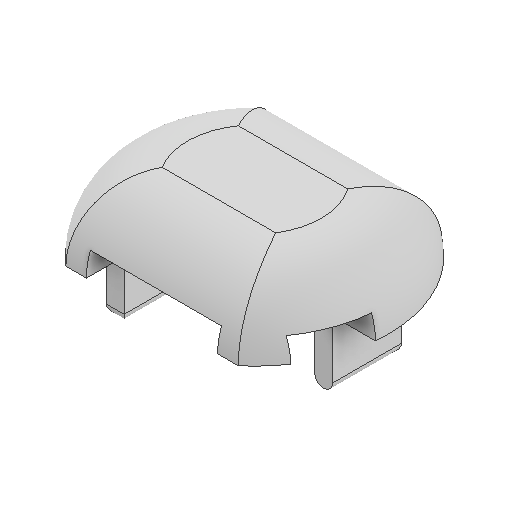
# Autodesk Inventor part: arm cover1
Saved by Autodesk Inventor 2025.2 (Build 292293000, 293)
## iProperties
Created: 2025-07-07
Part Number: arm cover1
Material: 일반
Document SubType Name: Modeling
Designer: joseph
Density: 1 g/cm^3
Appearance: 기본값
Author: joseph
Autodesk Inventor part; units mm, degrees
ref_plane "YZ Plane" through (0, 0, 0) normal (1, 0, 0) x (0, 1, 0)
ref_plane "XZ Plane" through (0, 0, 0) normal (0, 1, 0) x (-1, 0, 0)
ref_plane "XY Plane" through (0, 0, 0) normal (0, 0, 1) x (1, 0, 0)
sketch "스케치1" plane through (0, 0, 0) normal (0, 1, 0) x (-1, 0, 0)
  line L0 (14.7, -17.45) -> (14.7, -23.65)
  line L1 (-14.7, -23.65) -> (-14.7, -17.45)
  line L2 (-14.7, -17.45) -> (-20.25, -17.45)
  line L3 (-20.25, -17.45) -> (-20.25, 16.75)
  line L4 (-20.25, 16.75) -> (-14.7, 16.75)
  line L5 (-14.7, 16.75) -> (-14.7, 22.95)
  line L6 (14.7, 22.95) -> (14.7, 16.75)
  line L7 (14.7, 16.75) -> (20.45, 16.75)
  line L8 (20.45, 16.75) -> (20.45, -17.45)
  line L9 (20.45, -17.45) -> (14.7, -17.45)
  line L10 (-14.7, -23.65) -> (-18.4575, -23.65)
  line L11 (14.7, -23.65) -> (18.4575, -23.65)
  line L12 (14.7, 22.95) -> (19.3209, 22.95)
  line L13 (-14.7, 22.95) -> (-19.3209, 22.95)
  arc A0 (-19.3209, 22.95) -> (-18.4575, -23.65) centre (0, 0) ccw
  arc A1 (18.4575, -23.65) -> (19.3209, 22.95) centre (0, 0) ccw
  line L14 (-18.4575, -23.65) -> (-14.7, -23.65)
  line L15 (14.7, -23.65) -> (18.4575, -23.65)
  point P0 (-20, 0)
  point P1 (-30, 0)
  dimension "d12" = 40.7
  dimension "d13" = 34.2
  constraints: 32 end point, 4 point on circle, 2 centre point, 1 parallel, 1 point on line
  measures "d12" distance between parallel lines of L8 L3
  measures "d13" distance of L3.start L4.start
extrude "돌출1" add sketch "스케치1" along normal blind 5
sketch "스케치2" plane through (0, 5, 0) normal (0, 1, 0) x (1, 0, 0)
  line L0 (-14.7, 23.65) -> (-18.4575, 23.65) projected
  arc A0 (-18.4575, 23.65) -> (-19.3209, -22.95) centre (0, 0) ccw projected
  line L1 (-19.3209, -22.95) -> (-14.7, -22.95) projected
  line L2 (-14.7, -22.95) -> (-14.7, -16.75) projected
  line L3 (-14.7, -16.75) -> (-20.45, -16.75) projected
  line L4 (-20.45, -16.75) -> (-20.45, 17.45) projected
  line L5 (-20.45, 17.45) -> (-14.7, 17.45) projected
  line L6 (-14.7, 17.45) -> (-14.7, 23.65) projected
  line L7 (18.4575, 23.65) -> (14.7, 23.65) projected
  line L8 (14.7, 23.65) -> (14.7, 17.45) projected
  line L9 (14.7, 17.45) -> (20.25, 17.45) projected
  line L10 (20.25, 17.45) -> (20.25, -16.75) projected
  line L11 (20.25, -16.75) -> (14.7, -16.75) projected
  line L12 (14.7, -16.75) -> (14.7, -22.95) projected
  line L13 (14.7, -22.95) -> (19.3209, -22.95) projected
  arc A1 (19.3209, -22.95) -> (18.4575, 23.65) centre (0, 0) ccw projected
  line L14 (14.7, -22.95) -> (-14.7, -22.95)
  line L15 (-14.7, 23.65) -> (14.7, 23.65)
  constraints: 4 end point, 2 collinear
extrude "돌출2" add sketch "스케치2" along normal blind 10
fillet "모깎기1" radius 15 4 edges at (-29.9949, 15, -0.5558) (29.9949, 15, -0.5558) (0, 15, 22.95) (0, 15, -23.65)
sketch "스케치3" plane through (0, 5, 0) normal (0, -1, 0) x (1, 0, 0)
  line L0 (-14.7, 22.0921) -> (14.7, 22.0921) projected
  line L1 (-14.7, 22.0921) -> (-14.7, 16.75) projected
  line L2 (-14.7, 16.75) -> (-20.45, 16.75) projected
  line L3 (-20.45, 16.75) -> (-20.45, -17.45) projected
  line L4 (-20.45, -17.45) -> (-14.7, -17.45) projected
  line L5 (-14.7, -17.45) -> (-14.7, -22.7921) projected
  line L6 (14.7, -22.7921) -> (-14.7, -22.7921) projected
  line L7 (14.7, -22.7921) -> (14.7, -17.45) projected
  line L8 (14.7, -17.45) -> (20.25, -17.45) projected
  line L9 (20.25, -17.45) -> (20.25, 16.75) projected
  line L10 (20.25, 16.75) -> (14.7, 16.75) projected
  line L11 (14.7, 16.75) -> (14.7, 22.0921) projected
  line L12 (20.25, 16.75) -> (-20.45, 16.75)
  line L13 (-20.45, 16.75) -> (-20.45, 12.75)
  line L14 (-20.45, 12.75) -> (20.25, 12.75)
  line L15 (20.25, 12.75) -> (20.25, 16.75)
  line L16 (20.25, -17.45) -> (-20.45, -17.45)
  line L17 (-20.45, -17.45) -> (-20.45, -12.75)
  line L18 (-20.45, -12.75) -> (20.25, -12.75)
  line L19 (20.25, -12.75) -> (20.25, -17.45)
  line L20 (20.25, 12.75) -> (16.25, 12.75)
  line L21 (16.25, 12.75) -> (16.25, -12.75)
  line L22 (16.25, -12.75) -> (20.25, -12.75)
  line L23 (20.25, -12.75) -> (20.25, 12.75)
  line L24 (-20.45, 12.75) -> (-16.45, 12.75)
  line L25 (-16.45, 12.75) -> (-16.45, -12.75)
  line L26 (-16.45, -12.75) -> (-20.45, -12.75)
  line L27 (-20.45, -12.75) -> (-20.45, 12.75)
  point P0 (0, 0)
  point P1 (-16.45, 12.75)
  point P2 (20.25, -12.75)
  point P3 (20.25, 12.75)
  dimension "d5" = 4
  dimension "d6" = 4.7
  dimension "d7" = 4
  dimension "d8" = 4
  constraints: 32 end point, 8 parallel, 4 horizontal, 4 perpendicular, 4 point on line
  measures "d5" distance of L13.end L12.end
  measures "d6" distance of L16.end L17.end
  measures "d7" distance of L22.end L21.end
  measures "d8" distance of L25.end L26.end
extrude "돌출3" add sketch "스케치3" along normal blind 20 contours L14 L25 L18 L3 | L9 L18 L21 L14
fillet "모깎기2" radius 2 8 edges at (16.25, -15, 0) (18.25, -15, 12.75) (20.25, -15, 0) (18.25, -15, -12.75) (-16.45, -15, 0) (-18.45, -15, 12.75) (-20.45, -15, 0) (-18.45, -15, -12.75)
sketch "스케치4" plane through (16.25, 5, -12.75) normal (-1, 0, 0) x (0, 0, 1)
  line L0 (0, -18) -> (25.5, -18) projected
  line L1 (0, -5) -> (0, -18) projected
  line L2 (0, -5) -> (25.5, -5) projected
  line L3 (25.5, -5) -> (25.5, -18) projected
  line L4 (29.5, -5) -> (29.5, 0) projected
  line L5 (29.5, 0) -> (15.5, 0)
  line L6 (15.5, 0) -> (15.5, -23.2577)
  line L7 (15.5, -23.2577) -> (29.5, -23.2577)
  line L8 (29.5, -23.2577) -> (29.5, 0)
  point P0 (12.75, -5)
  dimension "d14" = 14
  constraints: 8 end point, 2 parallel, 1 horizontal, 1 perpendicular
  measures "d14" distance of L7.end L6.end
extrude "돌출4" cut sketch "스케치4" against normal blind 20 contours L6 L2 L3 L0 | L0 L3 L2 L6 L5 L4 L8 L7
